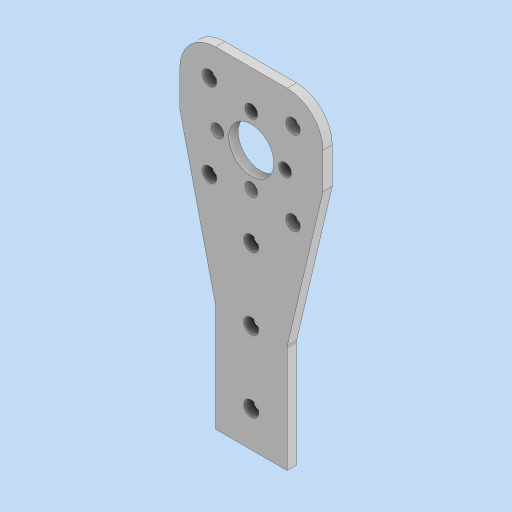
# Autodesk Inventor part: Arm Plate4
Saved by Autodesk Inventor 2024 (Build 280153000, 153)
## iProperties
Created: 2023-10-19
Part Number: Arm Plate4
Material: Generic
Document SubType Name: Modeling
Designer: ellen
Density: 1 g/cm^3
Appearance: Default
Author: ellen
Autodesk Inventor part; units mm, degrees
ref_plane "YZ Plane" through (0, 0, 0) normal (1, 0, 0) x (0, 1, 0)
ref_plane "XZ Plane" through (0, 0, 0) normal (0, 1, 0) x (-1, 0, 0)
ref_plane "XY Plane" through (0, 0, 0) normal (0, 0, 1) x (1, 0, 0)
sketch "Sketch1" plane through (0, 0, 0) normal (0, 0, 1) x (1, 0, 0)
  circle A0 centre (22.225, 53.975) radius 8
  circle A1 centre (22.225, 25.4) radius 2.6543
  circle A2 centre (22.225, 0) radius 2.6543
  line L0 (9.525, 0) -> (34.925, 0)
  circle A3 centre (22.225, -25.4) radius 2.6604
  line L1 (34.925, 0) -> (34.925, -38.1)
  line L2 (34.925, -38.1) -> (9.525, -38.1)
  line L3 (9.525, -38.1) -> (9.525, 0)
  circle A4 centre (10.225, 53.975) radius 2.2479
  circle A5 centre (22.225, 65.975) radius 2.2479
  circle A6 centre (22.225, 41.975) radius 2.2479
  circle A7 centre (34.225, 53.975) radius 2.2479
  circle A8 centre (22.225, 53.975) radius 20.955 construction
  circle A9 centre (7.4168, 39.1484) radius 2.5527
  circle A10 centre (37.0516, 39.1668) radius 2.5527
  circle A11 centre (37.0332, 68.8016) radius 2.5527
  circle A12 centre (7.3984, 68.7832) radius 2.5527
  line L4 (-3.175, 79.375) -> (47.625, 79.375)
  line L5 (-3.175, 79.375) -> (-3.175, 53.975)
  line L6 (-3.175, 53.975) -> (9.525, 0)
  line L7 (47.625, 79.375) -> (47.625, 53.975)
  line L8 (47.625, 53.975) -> (34.925, 0)
  point P0 (0, 0)
  point P1 (0, 53.975)
  point P2 (44.45, 53.975)
  point P3 (22.225, 76.2)
  point P4 (24.8793, 0)
  point P5 (19.5707, 0)
  point P6 (22.225, 0)
  point P7 (22.225, 79.375)
  dimension "d36" = 41.91
  dimension "d2" = 16
  dimension "d3" = 5.3086
  dimension "d4" = 5.3086
  dimension "d5" = 22.225
  dimension "d26" = 25.4
  dimension "d27" = 38.1
  dimension "d28" = 25.4
  dimension "d29" = 28.575
  dimension "d30" = 53.975
  dimension "d31" = 4.4958
  dimension "d32" = 12
  dimension "d33" = 12
  dimension "d34" = 12
  dimension "d35" = 12
  dimension "d37" = 5.1054
  dimension "d38" = 14.8082
  dimension "d41" = 360
  dimension "d43" = 50.8
  dimension "d44" = 0
  dimension "d45" = 25.4
  dimension "d46" = 25.4
  dimension "d47" = 25.4
  constraints: 18 end point, 12 centre point, 3 equal radius, 2 horizontal, 2 midpoint, 2 perpendicular, 2 vertical, 1 coincident, 1 parallel, 12 other
  measures "d2" diameter of A0
  measures "d3" diameter of A1
  measures "d4" diameter of A2
  measures "d5" distance of A0.centre point (22.225, 76.2)
  measures "d26" distance from line of A3.centre L0
  measures "d27" distance of L0.end L1.end
  measures "d28" distance of L1.end L2.end
  measures "d29" distance of A1.centre A0.centre
  measures "d30" distance of point (22.225, 0) A0.centre
  measures "d31" diameter of A4
  measures "d32" distance of A0.centre A4.centre
  measures "d33" distance of A7.centre A0.centre
  measures "d34" distance of A0.centre A5.centre
  measures "d35" distance of A0.centre A6.centre
  measures "d37" diameter of A9
  measures "d38" horizontal distance of A0.centre A9.centre
  measures "d43" distance of L4.start L4.end
  measures "d44" horizontal distance of A0.centre point (22.225, 79.375)
  measures "d45" distance of L4.start L5.end
  measures "d46" distance of L4.end L7.end
  measures "d47" distance from line of A0.centre L4
extrude "Extrusion1" add sketch "Sketch1" along normal blind 3.302 contours L0 L1 L2 L3 A2 | A2 L0 L6 L5 L4 L7 L8
fillet "Fillet13" radius 3.175 1 edges at (34.925, 0, 1.651)
fillet "Fillet14" radius 3.175 1 edges at (9.525, 0, 1.651)
fillet "Fillet15" radius 12.7 2 edges at (-3.175, 79.375, 1.651) (47.625, 79.375, 1.651)
body "Solid1"
